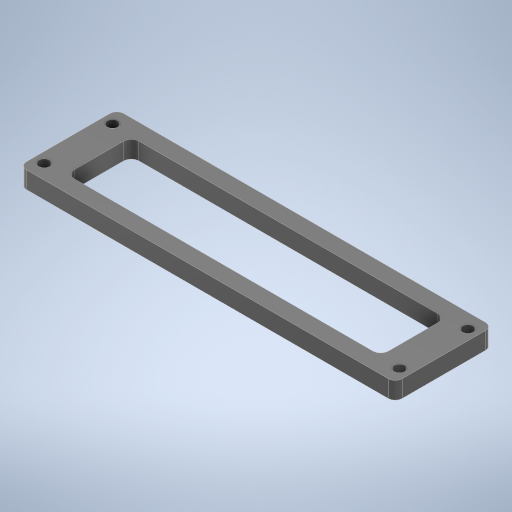
# Autodesk Inventor part: TorsoButtonLowerCoverFrame
Saved by Autodesk Inventor 2024.2 (Build 282272000, 272)
## iProperties
Created: 2024-06-13
Part Number: TorsoButtonLowerCoverFrame
Material: Acetal Resin, Black
Document SubType Name: Modeling
Designer: Masato Kubotera
Density: 1.425 g/cm^3
Appearance: Smooth - Black
Author: Masato Kubotera
Autodesk Inventor part; units mm, degrees
ref_plane "YZ Plane" through (0, 0, 0) normal (1, 0, 0) x (0, 1, 0)
ref_plane "XZ Plane" through (0, 0, 0) normal (0, 1, 0) x (-1, 0, 0)
ref_plane "XY Plane" through (0, 0, 0) normal (0, 0, 1) x (1, 0, 0)
derived "TorsoButtonUpperCoverFrame.ipt"
sketch "Sketch2" plane through (0, 0, 0) normal (0, 0, 1) x (1, 0, 0)
  line L0 (-41, 53) -> (-41, -53)
  arc A0 (-41, -53) -> (-39, -55) centre (-39, -53) ccw
  line L1 (-39, -55) -> (-14.5, -55)
  arc A1 (-14.5, -55) -> (-12.5, -53) centre (-14.5, -53) ccw
  line L2 (-12.5, -53) -> (-12.5, 53)
  arc A2 (-12.5, 53) -> (-14.5, 55) centre (-14.5, 53) ccw
  line L3 (-14.5, 55) -> (-39, 55)
  arc A3 (-39, 55) -> (-41, 53) centre (-39, 53) ccw
  line L4 (-16.25, 49.25) -> (-37.25, 49.25)
  line L5 (-39.5, 47) -> (-39.5, -47)
  line L6 (-37.25, -49.25) -> (-16.25, -49.25)
  line L7 (-14, -47) -> (-14, 47)
  line L8 (-14, 49.25) -> (-39.5, -49.25) construction
  line L9 (-39.5, 49.25) -> (-14, -49.25) construction
  line L10 (-16.25, 49) -> (-37.25, 49) construction
  arc A4 (-14.25, 47) -> (-16.25, 49) centre (-16.25, 47) ccw construction
  line L11 (-14.25, -47) -> (-14.25, 47) construction
  arc A5 (-16.25, -49) -> (-14.25, -47) centre (-16.25, -47) ccw construction
  line L12 (-37.25, -49) -> (-16.25, -49) construction
  arc A6 (-39.25, -47) -> (-37.25, -49) centre (-37.25, -47) ccw construction
  line L13 (-39.25, 47) -> (-39.25, -47) construction
  arc A7 (-37.25, 49) -> (-39.25, 47) centre (-37.25, 47) ccw construction
  arc A8 (-16.25, -49.25) -> (-14, -47) centre (-16.25, -47) ccw
  arc A9 (-14, 47) -> (-16.25, 49.25) centre (-16.25, 47) ccw
  arc A10 (-37.25, 49.25) -> (-39.5, 47) centre (-37.25, 47) ccw
  arc A11 (-39.5, -47) -> (-37.25, -49.25) centre (-37.25, -47) ccw
  line L14 (-36.5, -48.25) -> (-17, -48.25)
  line L15 (-15, -46.25) -> (-15, 46.25)
  line L16 (-17, 48.25) -> (-36.5, 48.25)
  line L17 (-38.5, 46.25) -> (-38.5, -46.25)
  line L18 (-38.5, -48.25) -> (-15, 48.25) construction
  line L19 (-15, -48.25) -> (-38.5, 48.25) construction
  arc A12 (-15, 46.25) -> (-17, 48.25) centre (-17, 46.25) ccw
  arc A13 (-36.5, 48.25) -> (-38.5, 46.25) centre (-36.5, 46.25) ccw
  arc A14 (-38.5, -46.25) -> (-36.5, -48.25) centre (-36.5, -46.25) ccw
  arc A15 (-17, -48.25) -> (-15, -46.25) centre (-17, -46.25) ccw
  line L20 (-35.75, -22.5) -> (-17.75, -22.5) construction
  line L21 (-17.75, -22.5) -> (-17.75, 22.5) construction
  line L22 (-35.75, 22.5) -> (-35.75, -22.5) construction
  line L23 (-17.75, 22.5) -> (-35.75, 22.5) construction
  point P0 (0, 0)
  point P1 (-36.75, 52)
  point P2 (-16.75, 52)
  point P3 (-16.75, -52)
  point P4 (-36.75, -52)
  point P5 (-26.75, 0)
  point P6 (-26.75, 0)
sketch "Sketch3" plane through (0, 0, 0) normal (0, 0, 1) x (1, 0, 0)
  line L0 (-34, -46) -> (-19.5, -46)
  line L1 (-17.25, -43.75) -> (-17.25, 43.75)
  line L2 (-19.5, 46) -> (-34, 46)
  line L3 (-36.25, 43.75) -> (-36.25, -43.75)
  line L4 (-36.25, -46) -> (-17.25, 46) construction
  line L5 (-17.25, -46) -> (-36.25, 46) construction
  line L6 (-39.25, 47) -> (-39.25, -47) construction
  line L7 (-37.25, -49) -> (-16.25, -49) construction
  arc A0 (-39.5, -47) -> (-37.25, -49.25) centre (-37.25, -47) ccw projected
  arc A1 (-36.25, -43.75) -> (-34, -46) centre (-34, -43.75) ccw
  arc A2 (-19.5, -46) -> (-17.25, -43.75) centre (-19.5, -43.75) ccw
  arc A3 (-17.25, 43.75) -> (-19.5, 46) centre (-19.5, 43.75) ccw
  arc A4 (-34, 46) -> (-36.25, 43.75) centre (-34, 43.75) ccw
  line L8 (-14.5, 55) -> (-39, 55) projected
  arc A5 (-39, 55) -> (-41, 53) centre (-39, 53) ccw projected
  line L9 (-41, 53) -> (-41, -53) projected
  arc A6 (-12.5, 53) -> (-14.5, 55) centre (-14.5, 53) ccw projected
  line L10 (-12.5, -53) -> (-12.5, 53) projected
  arc A7 (-14.5, -55) -> (-12.5, -53) centre (-14.5, -53) ccw projected
  line L11 (-39, -55) -> (-14.5, -55) projected
  arc A8 (-41, -53) -> (-39, -55) centre (-39, -53) ccw projected
  point P0 (0, 0)
  point P1 (-26.75, 0)
  point P2 (-26.75, 0)
  point P3 (-36.75, -52)
  point P4 (-16.75, -52)
  point P5 (-16.75, 52)
  point P6 (-36.75, 52)
  dimension "d1" = 3
  dimension "d2" = 3
  constraints: 12 end point, 8 point on circle, 8 point on line, 8 tangent, 4 centre point, 4 equal radius, 2 midpoint, 2 parallel, 1 coincident, 1 horizontal, 1 perpendicular
  measures "d1" distance between parallel lines of L3 L6
  measures "d2" distance between parallel lines of L7 L0
extrude "Extrusion1" add sketch "Sketch3" against normal blind 5
hole "Phi3.2" at (-36.75, -52, 0) at (-16.75, -52, 0) at (-36.75, 52, 0) at (-16.75, 52, 0) direction (0, 0, -1) diameter 3.2 end through all
equation "\"d2\" = d1"
body "Solid1"
